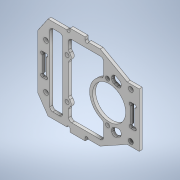
# Autodesk Inventor part: Trunk_neck_Lower_frame
Saved by Autodesk Inventor 2020.4 (Build 244396000, 396)
## iProperties
Created: 2022-01-02
Part Number: Trunk_neck_Lower_frame
Material: アルミニウム 2014-T4
Document SubType Name: Modeling
Designer: Masato Kubotera
Density: 2.8 g/cm^3
Appearance: 滑らか - 淡い灰色
Author: Masato Kubotera
Autodesk Inventor part; units mm, degrees
ref_plane "YZ Plane" through (0, 0, 0) normal (1, 0, 0) x (0, 1, 0)
ref_plane "XZ Plane" through (0, 0, 0) normal (0, 1, 0) x (-1, 0, 0)
ref_plane "XY Plane" through (0, 0, 0) normal (0, 0, 1) x (1, 0, 0)
sketch "スケッチ1" plane through (0, 0, 0) normal (0, 0, 1) x (1, 0, 0)
  circle A0 centre (0, 0) radius 10.5 construction
  line L0 (-28, -13.5) -> (-1, -13.5) construction
  line L1 (-1, -13.5) -> (-1, 13.5) construction
  line L2 (-1, 13.5) -> (-28, 13.5) construction
  line L3 (-28, 13.5) -> (-28, -13.5) construction
  line L4 (-28, -13.5) -> (-1, 13.5) construction
  line L5 (-1, -13.5) -> (-28, 13.5) construction
  line L6 (-31, -16) -> (12, -16) construction
  line L7 (12, -16) -> (12, 16) construction
  line L8 (12, 16) -> (-31, 16) construction
  line L9 (-31, 16) -> (-31, -16) construction
  line L10 (-31, -16) -> (12, 16) construction
  line L11 (12, -16) -> (-31, 16) construction
  line L12 (-31, -14.4) -> (-39.5, -14.4) construction
  line L13 (-39.5, -14.4) -> (-39.5, 14.4) construction
  line L14 (-39.5, 0) -> (12, 0) construction
  line L15 (-31, 14.4) -> (-39.5, 14.4) construction
  circle A1 centre (-1, -13.5) radius 1.35
  line L16 (-14.5, -13.5) -> (-14.5, 13.5) construction
  circle A2 centre (-28, -13.5) radius 1.35
  circle A3 centre (-1, 13.5) radius 1.35
  circle A4 centre (-28, 13.5) radius 1.35
  line L17 (14.5, -7.5) -> (17, -7.5) construction
  line L18 (17, -7.5) -> (17, 7.5) construction
  line L19 (17, 7.5) -> (14.5, 7.5) construction
  line L20 (14.5, 7.5) -> (14.5, -7.5) construction
  line L21 (14.5, -7.5) -> (17, 7.5) construction
  line L22 (17, -7.5) -> (14.5, 7.5) construction
  line L23 (14.45, 7.55) -> (17.05, 7.55)
  line L24 (17.05, 5.45) -> (17.05, -5.45)
  line L25 (17.05, -7.55) -> (14.45, -7.55)
  line L26 (14.45, -5.45) -> (14.45, 5.45)
  line L27 (14.45, 7.55) -> (17.05, -7.55) construction
  line L28 (17.05, 7.55) -> (14.45, -7.55) construction
  arc A5 (14.45, -5.45) -> (14.45, -7.55) centre (14.45, -6.5) ccw
  line L29 (15.75, -7.5) -> (15.75, 7.5) construction
  arc A6 (14.45, 7.55) -> (14.45, 5.45) centre (14.45, 6.5) ccw
  arc A7 (17.05, -7.55) -> (17.05, -5.45) centre (17.05, -6.5) ccw
  arc A8 (17.05, 5.45) -> (17.05, 7.55) centre (17.05, 6.5) ccw
  line L30 (-13.75, -16) -> (-13.75, 16) construction
  line L31 (-42, -7.5) -> (-44.5, -7.5) construction
  line L32 (-44.5, -7.5) -> (-44.5, 7.5) construction
  line L33 (-44.5, 7.5) -> (-42, 7.5) construction
  line L34 (-42, 7.5) -> (-42, -7.5) construction
  line L35 (-42, -7.5) -> (-44.5, 7.5) construction
  line L36 (-44.5, -7.5) -> (-42, 7.5) construction
  line L37 (-41.95, 7.55) -> (-44.55, 7.55)
  line L38 (-44.55, 5.45) -> (-44.55, -5.45)
  line L39 (-44.55, -7.55) -> (-41.95, -7.55)
  line L40 (-41.95, -5.45) -> (-41.95, 5.45)
  line L41 (-41.95, 7.55) -> (-44.55, -7.55) construction
  line L42 (-44.55, 7.55) -> (-41.95, -7.55) construction
  arc A9 (-41.95, -7.55) -> (-41.95, -5.45) centre (-41.95, -6.5) ccw
  line L43 (-43.25, -7.5) -> (-43.25, 7.5) construction
  arc A10 (-41.95, 5.45) -> (-41.95, 7.55) centre (-41.95, 6.5) ccw
  arc A11 (-44.55, -5.45) -> (-44.55, -7.55) centre (-44.55, -6.5) ccw
  arc A12 (-44.55, 7.55) -> (-44.55, 5.45) centre (-44.55, 6.5) ccw
  circle A13 centre (14.5, -15) radius 1.6
  circle A14 centre (14.5, 15) radius 1.6
  circle A15 centre (-42, -15) radius 1.6
  circle A16 centre (-42, 15) radius 1.6
  line L44 (12, -60.5) -> (17, -60.5) construction
  line L45 (17, -60.5) -> (17, 60.5) construction
  line L46 (17, 60.5) -> (12, 60.5) construction
  line L47 (12, -60.5) -> (17, 60.5) construction
  line L48 (17, -60.5) -> (12, 60.5) construction
  circle A17 centre (0, 0) radius 11
  arc A18 (-4.9833, 12.0069) -> (-4.9833, -12.0069) centre (0, 0) ccw
  line L49 (-3.75, -16) -> (1.75, -16) construction
  line L50 (1.75, -16) -> (1.75, 16) construction
  line L51 (1.75, 16) -> (-3.75, 16) construction
  line L52 (-3.75, 16) -> (-3.75, -16) construction
  line L53 (-3.75, -16) -> (1.75, 16) construction
  line L54 (1.75, -16) -> (-3.75, 16) construction
  line L55 (-39.5, -30) -> (12, -30) construction
  line L56 (-26, -30) -> (-16, -30)
  line L57 (-16, -30) -> (-16, -28)
  line L58 (-13.9, -28) -> (-6, -28)
  line L59 (20, -18) -> (20, 18)
  arc A19 (-13.9, -28) -> (-16, -28) centre (-14.95, -28) ccw
  line L60 (1.75, -14.5237) -> (1.75, -15.7196)
  line L61 (-21, -30) -> (-21, -25.7946) construction
  line L62 (-26, -30) -> (-26, -28)
  arc A20 (-26, -28) -> (-28.1, -28) centre (-27.05, -28) ccw
  line L63 (-39.5, -60.5) -> (-44.5, -60.5) construction
  line L64 (-44.5, -60.5) -> (-44.5, 60.5) construction
  line L65 (-44.5, 60.5) -> (-39.5, 60.5) construction
  line L66 (-39.5, 60.5) -> (-39.5, -60.5) construction
  line L67 (-47.5, -18) -> (-47.5, 18)
  line L68 (-26, 30) -> (-16, 30)
  line L69 (-16, 30) -> (-16, 28)
  arc A21 (-16, 28) -> (-13.9, 28) centre (-14.95, 28) ccw
  line L70 (-26, 30) -> (-26, 28)
  arc A22 (-28.1, 28) -> (-26, 28) centre (-27.05, 28) ccw
  line L71 (-37.5, -24) -> (-33, -24)
  line L72 (-33, 24) -> (-37.5, 24)
  line L73 (-39.5, 22) -> (-39.5, -22)
  line L74 (-39.5, -24) -> (-31, 24) construction
  line L75 (-31, -24) -> (-39.5, 24) construction
  arc A23 (-39.5, -22) -> (-37.5, -24) centre (-37.5, -22) ccw
  arc A24 (-33, -24) -> (-31, -22) centre (-33, -22) ccw
  arc A25 (-31, 22) -> (-33, 24) centre (-33, 22) ccw
  arc A26 (-37.5, 24) -> (-39.5, 22) centre (-37.5, 22) ccw
  line L76 (12, -60.5) -> (12, 60.5) construction
  arc A27 (3.25, -12.5872) -> (5.2, -11.9147) centre (0, 0) ccw
  arc A28 (3.25, -12.5872) -> (1.75, -14.5237) centre (3.75, -14.5237) ccw
  line L77 (-27, 9.8173) -> (-27, -9.8173)
  line L78 (-25, -24) -> (-5.75, -24)
  line L79 (-3.75, -22) -> (-3.75, -13.8542)
  line L80 (-31, -22) -> (-31, 22)
  arc A29 (-26.2632, -15.6321) -> (-26.2632, -11.3679) centre (-28, -13.5) ccw
  line L81 (-27, -17.1827) -> (-27, -22)
  line L82 (-25, 24) -> (-5.75, 24)
  line L83 (-3.75, 22) -> (-3.75, 13.8542)
  arc A30 (-26.2632, 11.3679) -> (-26.2632, 15.6321) centre (-28, 13.5) ccw
  line L84 (-27, 17.1827) -> (-27, 22)
  arc A31 (-27, -22) -> (-25, -24) centre (-25, -22) ccw
  arc A32 (-5.75, -24) -> (-3.75, -22) centre (-5.75, -22) ccw
  arc A33 (-3.75, -13.8542) -> (-4.9833, -12.0069) centre (-5.75, -13.8542) ccw
  arc A34 (-4.9833, 12.0069) -> (-3.75, 13.8542) centre (-5.75, 13.8542) ccw
  arc A35 (-3.75, 22) -> (-5.75, 24) centre (-5.75, 22) ccw
  arc A36 (-25, 24) -> (-27, 22) centre (-25, 22) ccw
  arc A37 (-27, 17.1827) -> (-26.2632, 15.6321) centre (-25, 17.1827) ccw
  arc A38 (-26.2632, 11.3679) -> (-27, 9.8173) centre (-25, 9.8173) ccw
  arc A39 (-26.2632, -15.6321) -> (-27, -17.1827) centre (-25, -17.1827) ccw
  arc A40 (-27, -9.8173) -> (-26.2632, -11.3679) centre (-25, -9.8173) ccw
  circle A41 centre (14.5, -15) radius 2.75 construction
  line L85 (12, -18) -> (20, -18)
  line L86 (-6, -28) -> (12, -18)
  line L87 (4.7213, -17.4679) -> (6.9713, -16.2179)
  line L88 (8, -14.4696) -> (8, -13.7477)
  line L89 (-47.5, -18) -> (-40.6672, -28)
  line L90 (-40.6672, -28) -> (-28.1, -28)
  arc A42 (1.75, -15.7196) -> (4.7213, -17.4679) centre (3.75, -15.7196) ccw
  arc A43 (8, -13.7477) -> (5.2, -11.9147) centre (6, -13.7477) ccw
  arc A44 (6.9713, -16.2179) -> (8, -14.4696) centre (6, -14.4696) ccw
  line L91 (-13.9, 28) -> (-6, 28)
  arc A45 (5.2, 11.9147) -> (3.25, 12.5872) centre (0, 0) ccw
  arc A46 (1.75, 14.5237) -> (3.25, 12.5872) centre (3.75, 14.5237) ccw
  line L92 (12, 18) -> (20, 18)
  line L93 (-6, 28) -> (12, 18)
  line L94 (4.7213, 17.4679) -> (6.9713, 16.2179)
  line L95 (8, 14.4696) -> (8, 13.7477)
  line L96 (-47.5, 18) -> (-40.6672, 28)
  line L97 (-40.6672, 28) -> (-28.1, 28)
  arc A47 (4.7213, 17.4679) -> (1.75, 15.7196) centre (3.75, 15.7196) ccw
  arc A48 (5.2, 11.9147) -> (8, 13.7477) centre (6, 13.7477) ccw
  arc A49 (8, 14.4696) -> (6.9713, 16.2179) centre (6, 14.4696) ccw
  line L98 (1.75, 14.5237) -> (1.75, 15.7196)
  point P0 (-14.5, 0)
  point P1 (-9.5, 0)
  point P2 (-14.5, 0)
  point P3 (15.75, 0)
  point P4 (15.75, 0)
  point P5 (15.75, 0)
  point P6 (15.75, 0)
  point P7 (-43.25, 0)
  point P8 (-43.25, 0)
  point P9 (-43.25, 0)
  point P10 (-43.25, 0)
  point P11 (14.5, 0)
  point P12 (14.5, 0)
  point P13 (-3.75, 12.4474)
  point P14 (-3.75, -12.4474)
  point P15 (-1, 0)
  point P16 (1.75, -12.8817)
  point P17 (20, 0)
  point P18 (-35.25, 0)
  point P19 (1.75, -19.1186)
  point P20 (8, -10.247)
  point P21 (-27, -24)
  point P22 (-3.75, -24)
  point P23 (-27, -16.0617)
  point P24 (-27, -10.9383)
  point P25 (-27, 24)
  point P26 (-3.75, 24)
  point P27 (-27, 16.0617)
  point P28 (-27, 10.9383)
  point P29 (-35.25, 0)
  dimension "d0" = 21
  dimension "d1" = 27
  dimension "d2" = 27
  dimension "d3" = 43
  dimension "d4" = 32
  dimension "d5" = 28.8
  dimension "d6" = 8.5
  dimension "d7" = 9.5
  dimension "d11" = 8.5
  dimension "d12" = 2.7
  dimension "d13" = 2.5
  dimension "d14" = 15
  dimension "d15" = 1.05
  dimension "d16" = 0.05
  dimension "d17" = 0.05
  dimension "d18" = 2.5
  dimension "d26" = 51.5
  dimension "d27" = 25.75
  dimension "d28" = 3.2
  dimension "d29" = 2.5
  dimension "d30" = 30
  dimension "d31" = 5
  dimension "d32" = 121
  dimension "d34" = 22
  dimension "d36" = 5.5
  dimension "d38" = 30.5
  dimension "d39" = 1.05
  dimension "d42" = 10
  dimension "d45" = 2
  dimension "d47" = 3
  dimension "d50" = 2
  dimension "d53" = 2
  dimension "d55" = 13
  dimension "d56" = 13
  dimension "d57" = 4
  dimension "d58" = 0
  dimension "d59" = 2.75
  dimension "d60" = 2
  dimension "d63" = 4
  dimension "d65" = 5.5
  dimension "d66" = 36
  dimension "d67" = 15
  dimension "d68" = 4
  dimension "d69" = 20
  dimension "d70" = 2
  dimension "d71" = 4
  dimension "d72" = 4
  constraints: 196 end point, 86 point on circle, 50 centre point, 38 point on line, 38 symmetric about line, 38 tangent, 35 midpoint, 34 vertical alignment, 25 equal radius, 16 perpendicular, 14 parallel, 9 horizontal, 7 coincident, 6 vertical, 3 collinear, 1 concentric, 22 other
  measures "d0" diameter of A0
  measures "d1" distance of L2.end L1.end
  measures "d2" distance of L1.end L0.end
  measures "d3" distance of L8.end L7.end
  measures "d4" distance of L7.end L6.end
  measures "d5" distance of L12.end L13.end
  measures "d6" distance of L12.start L12.end
  measures "d7" distance of point (0, 0) point (-9.5, 0)
  measures "d11" distance from line of L1 point (-9.5, 0)
  measures "d12" diameter of A1
  measures "d13" distance of L19.end L18.end
  measures "d14" distance of L18.end L17.end
  measures "d15" radius of A5
  measures "d16" distance between parallel lines of L26 L20
  measures "d17" distance between parallel lines of L25 L17
  measures "d18" distance between parallel lines of L20 L7
  measures "d26" horizontal distance of L6.end L12.end
  measures "d27" distance of L6.end L30.start
  measures "d28" diameter of A13
  measures "d29" horizontal distance of A13.centre L6.end
  measures "d30" distance of A14.centre A13.centre
  measures "d31" distance of L46.end L45.end
  measures "d32" distance of L45.end L44.end
  measures "d34" diameter of A17
  measures "d36" distance of L51.end L50.end
  measures "d38" distance between parallel lines of L44 L55
  measures "d39" radius of A19
  measures "d42" distance of L56.start L56.end
  measures "d45" distance between parallel lines of L55 L58
  measures "d47" distance from line of L59.start L45
  measures "d50" radius of A23
  measures "d53" radius of A28
  measures "d55" radius of A18
  measures "d56" radius of A27
  measures "d57" distance between parallel lines of L77 L9
  measures "d58" distance from line of L80 L6.start
  measures "d59" radius of A29
  measures "d60" radius of A31
  measures "d63" distance between parallel lines of L78 L58
  measures "d65" diameter of A41
  measures "d66" distance of L59.start L59.end
  measures "d67" horizontal distance of L58.end L61.start
  measures "d68" distance edge to line of A23 L89
  measures "d69" horizontal distance of L61.start point (-1, 0)
  measures "d70" radius of A42
  measures "d71" distance between parallel lines of L86 L87
  measures "d72" distance between parallel lines of L76 L88
extrude "押し出し1" add sketch "スケッチ1" along normal blind 2
equation "\"d17\" = d16"
equation "\"d27\" = 0.5 * d26"
equation "\"d39\" = d15"
